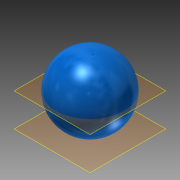
# Autodesk Inventor part: JLF-TP-8YT_ball
Saved by Autodesk Inventor 2013 (Build 170138000, 138)
## iProperties
Created: 2013-01-27
Part Number: JLF-TP-8YT_ball
Material: Acrylic, Clear(1)
Document SubType Name: Modeling
Designer: xylzlyx
Density: 1 g/cm^3
Author: xylzlyx
Autodesk Inventor part; units mm, degrees
ref_plane "YZ Plane" through (0, 0, 0) normal (1, 0, 0) x (0, 1, 0)
ref_plane "XZ Plane" through (0, 0, 0) normal (0, 1, 0) x (-1, 0, 0)
sketch "Sketch1" plane through (0, 0, 0) normal (0, 0, 1) x (1, 0, 0)
  circle A0 centre (0, 0) radius 18
  line L0 (-18, 0) -> (18, 0)
  dimension "d0" = 36
  dimension "d1" = 36
  constraints: 2 end point, 2 point on circle, 1 centre point, 1 coincident, 1 horizontal
  measures "d0" diameter of A0
  measures "d1" distance of L0.start L0.end
revolve "Ball" add sketch "Sketch1" angle 360 about axis through (-18, 0, 0) along (1, 0, 0) picked at (3.4084, 4.9379) contours L0 A0
ref_plane "BottomCuttingPlane" through (0, 0, -17.25) normal (0, 0, 1) x (1, 0, 0)
sketch "CutBottomSketch" plane through (0, 0, -17.25) normal (0, 0, 1) x (1, 0, 0)
  circle A0 centre (0, 0) radius 5.1417 projected
extrude "FlattenBottom" cut sketch "CutBottomSketch" against normal blind 10
sketch "Anchor" plane through (0, 0, -17.25) normal (0, 0, -1) x (-1, 0, 0)
  circle A0 centre (0, 0) radius 5.1417 projected
  circle A1 centre (0, 0) radius 4
  circle A2 centre (0, 0) radius 2.5
  dimension "d6" = 8
  dimension "d7" = 5
  constraints: 2 centre point, 2 coincident
  measures "d6" diameter of A1
  measures "d7" diameter of A2
extrude "Extrusion2" cut sketch "Anchor" against normal blind 10 contours A2
thread "Thread1" size "M5x0.8" class "6H" standard "ANSI Metric M Profile" full length
body "Solid1"
